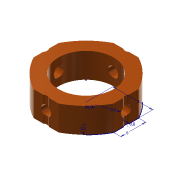
# Autodesk Inventor part: orthogonalize_block
Saved by Autodesk Inventor 2018 (Build 220112000, 112)
## iProperties
Created: 2018-08-31
Part Number: orthogonalize_block
Material: 一般
Document SubType Name: Modeling
Designer: student
Density: 1 g/cm^3
Appearance: 滑らか - 淡いオレンジ
Author: student
Autodesk Inventor part; units mm, degrees
ref_plane "YZ Plane" through (0, 0, 0) normal (1, 0, 0) x (0, 1, 0)
ref_plane "XZ Plane" through (0, 0, 0) normal (0, 1, 0) x (-1, 0, 0)
ref_plane "XY Plane" through (0, 0, 0) normal (0, 0, 1) x (1, 0, 0)
sketch "スケッチ1" plane through (0, 0, 0) normal (0, 0, 1) x (1, 0, 0)
  arc A0 (3.8891, -3.8891) -> (3.8891, 3.8891) centre (0, 0) ccw
  line L0 (8, 2.5) -> (8, 0.6)
  arc A1 (8, 0.6) -> (8, -0.6) centre (8.8, 0) ccw
  line L1 (7.8, 0) -> (8.8, 0) construction
  line L2 (0, 0) -> (3.8891, 3.8891) construction
  line L3 (5.6569, 5.6569) -> (3.8891, 3.8891)
  line L4 (0, 0) -> (3.8891, -3.8891) construction
  line L5 (0, 0) -> (5.5, 0) construction
  line L6 (3.8891, -3.8891) -> (5.6569, -5.6569)
  line L7 (8, -0.6) -> (8, -2.5)
  arc A2 (5.6569, -5.6569) -> (8, -2.5) centre (-3.8404, 3.8404) ccw
  arc A3 (8, 2.5) -> (5.6569, 5.6569) centre (-3.8404, -3.8404) ccw
  dimension "d5" = 0.8
  dimension "d9" = 90
  dimension "d10" = 1
  dimension "d11" = 8
  dimension "d12" = 5.5
  dimension "d14" = 5
  dimension "d21" = 2.5
  constraints: 16 end point, 10 point on circle, 4 centre point, 3 point on line, 3 symmetric about line, 2 coincident, 2 collinear, 2 horizontal, 2 vertical, 1 equal radius
  measures "d5" distance from line of L0 L1.end
  measures "d9" angle of L4 L2
  measures "d10" radius of A1
  measures "d11" distance from line of point (0, 0) L0
  measures "d12" radius of A0
  measures "d14" distance of L7.end L0.start
  measures "d21" distance of L4.end L6.end
extrude "押し出し1" add sketch "スケッチ1" along normal blind 5
sketch "スケッチ2" plane through (8, -2.5, 0) normal (1, 0, 0) x (0, 0, -1)
  line L0 (0, 2.5) -> (-5, 2.5) construction
  line L1 (-5, 1.9) -> (-5, 3.1) construction
  circle A0 centre (-2.5, 2.5) radius 1
  dimension "d15" = 2
  constraints: 2 end point, 2 midpoint, 1 centre point
  measures "d15" diameter of A0
extrude "押し出し2" cut sketch "スケッチ2" against normal blind 5
pattern_circular "円形状パターン1" count 4 over 360 about axis through (0, 0, -10) along (0, 0, 1) of "押し出し1", "押し出し2"
